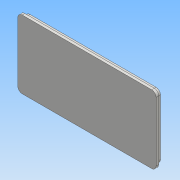
# Autodesk Inventor part: Box2_bottom
Saved by Autodesk Inventor 2016 (Build 200138000, 138)
## iProperties
Created: 2015-09-13
Part Number: Box2_bottom
Material: PPS Plastic
Document SubType Name: Modeling
Designer: Openlab
Density: 1.637 g/cm^3
Appearance: White
Author: Openlab
Autodesk Inventor part; units mm, degrees
ref_plane "YZ Plane" through (0, 0, 0) normal (1, 0, 0) x (0, 1, 0)
ref_plane "XZ Plane" through (0, 0, 0) normal (0, 1, 0) x (-1, 0, 0)
ref_plane "XY Plane" through (0, 0, 0) normal (0, 0, 1) x (1, 0, 0)
sketch "Sketch1" plane through (0, 0, 0) normal (0, 1, 0) x (-1, 0, 0)
  line L0 (-70, 35) -> (70, 35)
  line L1 (75, 30) -> (75, -30)
  line L2 (70, -35) -> (-70, -35)
  line L3 (-75, -30) -> (-75, 30)
  line L4 (-75, 35) -> (75, -35) construction
  line L5 (75, 35) -> (-75, -35) construction
  arc A0 (75, 30) -> (70, 35) centre (70, 30) ccw
  arc A1 (70, -35) -> (75, -30) centre (70, -30) ccw
  arc A2 (-70, 35) -> (-75, 30) centre (-70, 30) ccw
  arc A3 (-75, -30) -> (-70, -35) centre (-70, -30) ccw
  line L6 (-72, 37) -> (72, 37)
  line L7 (77, 32) -> (77, -32)
  line L8 (72, -37) -> (-72, -37)
  line L9 (-77, -32) -> (-77, 32)
  line L10 (-77, 37) -> (77, -37) construction
  line L11 (77, 37) -> (-77, -37) construction
  arc A4 (77, 32) -> (72, 37) centre (72, 32) ccw
  arc A5 (72, -37) -> (77, -32) centre (72, -32) ccw
  arc A6 (-77, -32) -> (-72, -37) centre (-72, -32) ccw
  arc A7 (-72, 37) -> (-77, 32) centre (-72, 32) ccw
  line L12 (74, 39) -> (-74, 39)
  line L13 (-79, 34) -> (-79, -34)
  line L14 (-74, -39) -> (74, -39)
  line L15 (79, -34) -> (79, 34)
  line L16 (79, 39) -> (-79, -39) construction
  line L17 (-79, 39) -> (79, -39) construction
  arc A8 (79, 34) -> (74, 39) centre (74, 34) ccw
  arc A9 (-74, 39) -> (-79, 34) centre (-74, 34) ccw
  arc A10 (-79, -34) -> (-74, -39) centre (-74, -34) ccw
  arc A11 (74, -39) -> (79, -34) centre (74, -34) ccw
  line L18 (-22.75, 23.25) -> (-35.25, 23.25) construction
  line L19 (-35.25, 23.25) -> (-35.25, 19) construction
  line L20 (-35.25, 10.75) -> (-22.75, 10.75) construction
  line L21 (-22.75, 10.75) -> (-22.75, 15) construction
  line L22 (56.9183, 17) -> (21.35, 17) construction
  line L23 (40.8, -24) -> (40.8, -20.1) construction
  line L24 (-55.8, 24) -> (-55.8, 12) construction
  line L25 (-20.25, 15.5) -> (-22.25, 15.5) construction
  line L26 (-22.25, 18.5) -> (-20.25, 18.5) construction
  line L27 (-35.75, 15.5) -> (-37.75, 15.5) construction
  line L28 (-37.75, 18.5) -> (-35.75, 18.5) construction
  line L29 (-40.55, 18.5) -> (-53.5, 18.5) construction
  line L30 (-40.55, 15.5) -> (-53.5, 15.5) construction
  line L31 (-60, 8.5) -> (45, 8.5) construction
  line L32 (38.5, 20.5) -> (37, 20.5) construction
  line L33 (37, 13.5) -> (38.5, 13.5) construction
  line L34 (-60, 5) -> (-60, -25) construction
  line L35 (21.35, -8.5) -> (45, -8.5) construction
  line L36 (-29, 20.0147) -> (-29, -25.5) construction
  line L37 (31.2062, 0) -> (-4.2501, 0) construction
  line L38 (-35.25, 6.25) -> (-35.25, 2) construction
  line L39 (-22.75, 6.25) -> (-35.25, 6.25) construction
  line L40 (-22.75, -6.25) -> (-22.75, -2) construction
  line L41 (-35.25, -6.25) -> (-22.75, -6.25) construction
  line L42 (-22.25, 1.5) -> (-20.25, 1.5) construction
  line L43 (-20.25, -1.5) -> (-22.25, -1.5) construction
  line L44 (38.5, 3.5) -> (37, 3.5) construction
  line L45 (37, -3.5) -> (38.5, -3.5) construction
  line L46 (-22.75, -10.75) -> (-35.25, -10.75) construction
  line L47 (-22.75, -23.25) -> (-22.75, -19) construction
  line L48 (-35.25, -23.25) -> (-22.75, -23.25) construction
  line L49 (56.3008, -17) -> (21.35, -17) construction
  line L50 (38.5, -13.5) -> (37, -13.5) construction
  line L51 (37, -20.5) -> (38.5, -20.5) construction
  line L52 (-20.25, -18.5) -> (-22.25, -18.5) construction
  line L53 (44.5, 5.5) -> (43.5, 5.5) construction
  line L54 (41.3, 11.5) -> (43.5, 11.5) construction
  line L55 (-37.75, -15.5) -> (-35.75, -15.5) construction
  line L56 (-35.75, -18.5) -> (-37.75, -18.5) construction
  line L57 (-40.55, -18.5) -> (-53.5, -18.5) construction
  line L58 (-37.75, 1.5) -> (-35.75, 1.5) construction
  line L59 (-35.75, -1.5) -> (-37.75, -1.5) construction
  line L60 (-40.55, -1.5) -> (-53.5, -1.5) construction
  line L61 (-58.5, 5.5) -> (-59.5, 5.5) construction
  line L62 (-59.5, 11.5) -> (-58.5, 11.5) construction
  line L63 (38.5, 5.5) -> (37, 5.5) construction
  line L64 (37, 5.5) -> (37, 11.5) construction
  line L65 (37, 11.5) -> (38.5, 11.5) construction
  line L66 (-53.5, 5.5) -> (-52.5, 5.5) construction
  line L67 (-52.5, 5.5) -> (-52.5, 11.5) construction
  line L68 (-52.5, 11.5) -> (-53.5, 11.5) construction
  line L69 (-54, 24) -> (-54, 19) construction
  line L70 (-54, 5) -> (-54, 2) construction
  arc A12 (-12.95, 13.5) -> (-12.95, 3.5) centre (-12.95, 8.5) ccw construction
  arc A13 (31, 3.5) -> (31, 13.5) centre (31, 8.5) ccw construction
  arc A14 (-12.95, -3.5) -> (-12.95, -13.5) centre (-12.95, -8.5) ccw construction
  arc A15 (31, -13.5) -> (31, -3.5) centre (31, -8.5) ccw construction
  line L71 (-12.95, 13.5) -> (31, 13.5) construction
  line L72 (-12.95, 3.5) -> (31, 3.5) construction
  line L73 (-12.95, -3.5) -> (31, -3.5) construction
  line L74 (-12.95, -13.5) -> (31, -13.5) construction
  arc A16 (-45.05, -13.5) -> (-45.05, -3.5) centre (-45.05, -8.5) ccw construction
  line L75 (43.5, -24) -> (43.5, -19.6) construction
  line L76 (-58.5, 24) -> (-58.5, 11.5) construction
  arc A17 (-46, -3.5) -> (-46, -13.5) centre (-46, -8.5) ccw construction
  arc A18 (-46, 13.5) -> (-46, 3.5) centre (-46, 8.5) ccw construction
  line L77 (-45.05, -13.5) -> (-46, -13.5) construction
  line L78 (-46, -3.5) -> (-45.05, -3.5) construction
  line L79 (-46, 3.5) -> (-45.05, 3.5) construction
  line L80 (-45.05, 13.5) -> (-46, 13.5) construction
  arc A19 (-45.05, 3.5) -> (-45.05, 13.5) centre (-45.05, 8.5) ccw construction
  line L81 (29.8763, -15.5) -> (-17.45, -15.5) construction
  line L82 (29.8763, -18.5) -> (-17.45, -18.5) construction
  line L83 (29.8763, -1.5) -> (-17.45, -1.5) construction
  line L84 (29.8763, 1.5) -> (-17.45, 1.5) construction
  line L85 (29.8763, 15.5) -> (-17.45, 15.5) construction
  line L86 (29.8763, 18.5) -> (-17.45, 18.5) construction
  arc A20 (32, -14.4) -> (29.8763, -15.5) centre (32, -17) ccw construction
  arc A21 (29.8763, -18.5) -> (32, -19.6) centre (32, -17) ccw construction
  arc A22 (32, 2.6) -> (29.8763, 1.5) centre (32, 0) ccw construction
  arc A23 (29.8763, -1.5) -> (32, -2.6) centre (32, 0) ccw construction
  arc A24 (32, 19.6) -> (29.8763, 18.5) centre (32, 17) ccw construction
  arc A25 (29.8763, 15.5) -> (32, 14.4) centre (32, 17) ccw construction
  arc A26 (34.4725, -25.0625) -> (31, -22) centre (31, -25.5) ccw construction
  arc A27 (-12.95, -22) -> (-16.4225, -25.0625) centre (-12.95, -25.5) ccw construction
  arc A28 (35.7697, -24) -> (31, -20.5) centre (31, -25.5) ccw construction
  line L87 (31, -20.5) -> (-12.95, -20.5) construction
  line L88 (34.9686, -25.5) -> (44.5, -25.5) construction
  line L89 (31, -22) -> (-12.95, -22) construction
  arc A29 (-12.95, -20.5) -> (-17.7197, -24) centre (-12.95, -25.5) ccw construction
  arc A30 (-17.6941, 23.9209) -> (-12.95, 20.5) centre (-12.95, 25.5) ccw construction
  arc A31 (-16.4225, 25.0625) -> (-12.95, 22) centre (-12.95, 25.5) ccw construction
  line L90 (31, 22) -> (-12.95, 22) construction
  line L91 (31, 20.5) -> (-12.95, 20.5) construction
  line L92 (35.7697, 24) -> (40.8, 24) construction
  line L93 (44.5, 25.5) -> (34.9686, 25.5) construction
  arc A32 (31, 22) -> (34.4725, 25.0625) centre (31, 25.5) ccw construction
  arc A33 (31, 20.5) -> (35.7697, 24) centre (31, 25.5) ccw construction
  arc A34 (-41.5775, -25.0625) -> (-45.05, -22) centre (-45.05, -25.5) ccw construction
  arc A35 (-46, -22) -> (-49.4725, -25.0625) centre (-46, -25.5) ccw construction
  line L94 (-45.05, -20.5) -> (-46, -20.5) construction
  line L95 (-45.05, -22) -> (-46, -22) construction
  arc A36 (-46, -20.5) -> (-50.7697, -24) centre (-46, -25.5) ccw construction
  arc A37 (-40.2803, -24) -> (-45.05, -20.5) centre (-45.05, -25.5) ccw construction
  line L96 (-17.7197, -24) -> (-40.2803, -24) construction
  line L97 (-50.7697, -24) -> (-58.5, -24) construction
  line L98 (-59.5, -25.5) -> (-49.9686, -25.5) construction
  line L99 (-17.2197, -25.5) -> (-16.9186, -25.5) construction
  line L100 (-45.05, 20.5) -> (-46, 20.5) construction
  line L101 (-45.05, 22) -> (-46, 22) construction
  arc A38 (-49.4725, 25.0625) -> (-46, 22) centre (-46, 25.5) ccw construction
  arc A39 (-45.05, 22) -> (-41.5775, 25.0625) centre (-45.05, 25.5) ccw construction
  arc A40 (-50.7697, 24) -> (-46, 20.5) centre (-46, 25.5) ccw construction
  arc A41 (-45.05, 20.5) -> (-40.336, 23.8333) centre (-45.05, 25.5) ccw construction
  line L102 (-16.9186, 25.5) -> (-17.2197, 25.5) construction
  line L103 (-49.9686, 25.5) -> (-59.5, 25.5) construction
  line L104 (-58.5, 24) -> (-50.7697, 24) construction
  line L105 (-40.3074, 24) -> (-17.7197, 24) construction
  line L106 (-17.7197, -24) -> (-17.7197, -25) construction
  line L107 (-40.2803, -24) -> (-40.2803, -25) construction
  line L108 (-40.3074, 24) -> (-40.3074, 25) construction
  line L109 (-17.7197, 24.0788) -> (-17.7197, 25) construction
  line L110 (43.5, 11.5) -> (44.5, 11.5) construction
  line L111 (43.5, 5.5) -> (41.3, 5.5) construction
  line L112 (-56.3, 11.5) -> (-58.5, 11.5) construction
  line L113 (-56.3, 5.5) -> (-58.5, 5.5) construction
  line L114 (-17.95, -21) -> (-19.75, -21) construction
  line L115 (-19.75, -13) -> (-17.95, -13) construction
  line L116 (-17.95, -4) -> (-19.75, -4) construction
  line L117 (-19.75, 4) -> (-17.95, 4) construction
  line L118 (-17.95, 13) -> (-19.75, 13) construction
  line L119 (-19.75, 21) -> (-17.95, 21) construction
  line L120 (-38.25, -21) -> (-40.05, -21) construction
  line L121 (-40.05, -13) -> (-38.25, -13) construction
  line L122 (-38.25, -4) -> (-40.05, -4) construction
  line L123 (-40.05, 4) -> (-38.25, 4) construction
  line L124 (-38.25, 13) -> (-40.05, 13) construction
  line L125 (-40.05, 21) -> (-38.25, 21) construction
  line L126 (-17.95, -13) -> (-17.95, -15) construction
  line L127 (-17.95, -19) -> (-17.95, -21) construction
  line L128 (-19.75, -21) -> (-19.75, -19) construction
  line L129 (-17.95, 4) -> (-17.95, 2) construction
  line L130 (-17.95, -2) -> (-17.95, -4) construction
  line L131 (-19.75, -4) -> (-19.75, -2) construction
  line L132 (-19.75, 2) -> (-19.75, 4) construction
  line L133 (-17.95, 21) -> (-17.95, 19) construction
  line L134 (-17.95, 15) -> (-17.95, 13) construction
  line L135 (-19.75, 13) -> (-19.75, 15) construction
  line L136 (-19.75, 19) -> (-19.75, 21) construction
  line L137 (-38.25, -13) -> (-38.25, -15) construction
  line L138 (-38.25, -19) -> (-38.25, -21) construction
  line L139 (-40.05, -21) -> (-40.05, -19) construction
  line L140 (-40.05, -15) -> (-40.05, -13) construction
  line L141 (-38.25, 4) -> (-38.25, 2) construction
  line L142 (-38.25, -2) -> (-38.25, -4) construction
  line L143 (-40.05, -4) -> (-40.05, -2) construction
  line L144 (-40.05, 2) -> (-40.05, 4) construction
  line L145 (-38.25, 21) -> (-38.25, 19) construction
  line L146 (-38.25, 15) -> (-38.25, 13) construction
  line L147 (-40.05, 13) -> (-40.05, 15) construction
  line L148 (-40.05, 19) -> (-40.05, 21) construction
  line L149 (38.5, -11.5) -> (37, -11.5) construction
  line L150 (37, -11.5) -> (37, -5.5) construction
  line L151 (37, -5.5) -> (38.5, -5.5) construction
  line L152 (39, -21) -> (39, -24) construction
  arc A42 (-19.75, -19) -> (-20.25, -18.5) centre (-20.25, -19) ccw construction
  arc A43 (-17.45, -18.5) -> (-17.95, -19) centre (-17.45, -19) ccw construction
  arc A44 (-19.75, -2) -> (-20.25, -1.5) centre (-20.25, -2) ccw construction
  arc A45 (-17.45, -1.5) -> (-17.95, -2) centre (-17.45, -2) ccw construction
  arc A46 (-17.95, 2) -> (-17.45, 1.5) centre (-17.45, 2) ccw construction
  arc A47 (-20.25, 1.5) -> (-19.75, 2) centre (-20.25, 2) ccw construction
  arc A48 (-19.75, 15) -> (-20.25, 15.5) centre (-20.25, 15) ccw construction
  arc A49 (-17.45, 15.5) -> (-17.95, 15) centre (-17.45, 15) ccw construction
  arc A50 (-17.95, 19) -> (-17.45, 18.5) centre (-17.45, 19) ccw construction
  arc A51 (-20.25, 18.5) -> (-19.75, 19) centre (-20.25, 19) ccw construction
  arc A52 (-38.25, 19) -> (-37.75, 18.5) centre (-37.75, 19) ccw construction
  arc A53 (-40.55, 18.5) -> (-40.05, 19) centre (-40.55, 19) ccw construction
  arc A54 (-40.05, 15) -> (-40.55, 15.5) centre (-40.55, 15) ccw construction
  arc A55 (-37.75, 15.5) -> (-38.25, 15) centre (-37.75, 15) ccw construction
  arc A56 (-38.25, 2) -> (-37.75, 1.5) centre (-37.75, 2) ccw construction
  arc A57 (-40.55, 1.5) -> (-40.05, 2) centre (-40.55, 2) ccw construction
  arc A58 (-40.05, -2) -> (-40.55, -1.5) centre (-40.55, -2) ccw construction
  arc A59 (-37.75, -1.5) -> (-38.25, -2) centre (-37.75, -2) ccw construction
  arc A60 (-38.25, -15) -> (-37.75, -15.5) centre (-37.75, -15) ccw construction
  arc A61 (-40.55, -15.5) -> (-40.05, -15) centre (-40.55, -15) ccw construction
  arc A62 (-37.75, -18.5) -> (-38.25, -19) centre (-37.75, -19) ccw construction
  arc A63 (-40.05, -19) -> (-40.55, -18.5) centre (-40.55, -19) ccw construction
  line L153 (36.5, -19.6) -> (32, -19.6) construction
  line L154 (37, -13.5) -> (37, -13.9) construction
  line L155 (32, -14.4) -> (36.5, -14.4) construction
  line L156 (36.5, -2.6) -> (32, -2.6) construction
  line L157 (37, 3.5) -> (37, 3.1) construction
  line L158 (37, -3.1) -> (37, -3.5) construction
  line L159 (32, 2.6) -> (36.5, 2.6) construction
  line L160 (36.5, 14.4) -> (32, 14.4) construction
  line L161 (37, 20.5) -> (37, 20.1) construction
  line L162 (37, 13.9) -> (37, 13.5) construction
  line L163 (32, 19.6) -> (36.5, 19.6) construction
  arc A64 (36.5, -14.4) -> (37, -13.9) centre (36.5, -13.9) ccw construction
  arc A65 (39, -12) -> (38.5, -11.5) centre (38.5, -12) ccw construction
  arc A66 (38.5, -5.5) -> (39, -5) centre (38.5, -5) ccw construction
  arc A67 (39, 5) -> (38.5, 5.5) centre (38.5, 5) ccw construction
  arc A68 (38.5, 11.5) -> (39, 12) centre (38.5, 12) ccw construction
  arc A69 (37, -3.1) -> (36.5, -2.6) centre (36.5, -3.1) ccw construction
  arc A70 (36.5, 2.6) -> (37, 3.1) centre (36.5, 3.1) ccw construction
  arc A71 (37, 13.9) -> (36.5, 14.4) centre (36.5, 13.9) ccw construction
  arc A72 (36.5, 19.6) -> (37, 20.1) centre (36.5, 20.1) ccw construction
  line L164 (43.5, -2.6) -> (43.5, 2.6) construction
  line L165 (43.5, -2.6) -> (41.3, -2.6) construction
  line L166 (37, -20.5) -> (37, -20.1) construction
  arc A73 (37, -20.1) -> (36.5, -19.6) centre (36.5, -20.1) ccw construction
  line L167 (39, -13) -> (39, -12) construction
  line L168 (39, 4) -> (39, 5) construction
  line L169 (39, 21) -> (39, 24) construction
  line L170 (43.5, -19.6) -> (43.5, -14.4) construction
  line L171 (43.5, -19.6) -> (41.3, -19.6) construction
  line L172 (43.5, -24) -> (40.8, -24) construction
  line L173 (40.8, -24) -> (39, -24) construction
  line L174 (39, -24) -> (35.7697, -24) construction
  line L175 (41.3, -14.4) -> (43.5, -14.4) construction
  line L176 (43.5, -14.4) -> (43.5, -2.6) construction
  line L177 (40.8, -13.9) -> (40.8, -3.1) construction
  line L178 (39, -4) -> (39, -5) construction
  line L179 (43.5, 2.6) -> (43.5, 5.5) construction
  line L180 (41.3, 2.6) -> (43.5, 2.6) construction
  line L181 (40.8, 3.1) -> (40.8, 5) construction
  line L182 (43.5, 14.4) -> (43.5, 19.6) construction
  line L183 (43.5, 14.4) -> (41.3, 14.4) construction
  line L184 (45, -25) -> (45, 5) construction
  line L185 (43.5, 19.6) -> (43.5, 24) construction
  line L186 (40.8, 20.1) -> (40.8, 24) construction
  line L187 (41.3, 19.6) -> (43.5, 19.6) construction
  line L188 (43.5, 11.5) -> (43.5, 14.4) construction
  line L189 (40.8, 24) -> (43.5, 24) construction
  line L190 (40.8, 12) -> (40.8, 13.9) construction
  line L191 (39, 13) -> (39, 12) construction
  arc A74 (38.5, -13.5) -> (39, -13) centre (38.5, -13) ccw construction
  arc A75 (39, -4) -> (38.5, -3.5) centre (38.5, -4) ccw construction
  arc A76 (38.5, 3.5) -> (39, 4) centre (38.5, 4) ccw construction
  arc A77 (39, 13) -> (38.5, 13.5) centre (38.5, 13) ccw construction
  arc A78 (38.5, 20.5) -> (39, 21) centre (38.5, 21) ccw construction
  arc A79 (41.3, -19.6) -> (40.8, -20.1) centre (41.3, -20.1) ccw construction
  arc A80 (40.8, -13.9) -> (41.3, -14.4) centre (41.3, -13.9) ccw construction
  arc A81 (41.3, -2.6) -> (40.8, -3.1) centre (41.3, -3.1) ccw construction
  arc A82 (40.8, 3.1) -> (41.3, 2.6) centre (41.3, 3.1) ccw construction
  arc A83 (41.3, 14.4) -> (40.8, 13.9) centre (41.3, 13.9) ccw construction
  arc A84 (40.8, 20.1) -> (41.3, 19.6) centre (41.3, 20.1) ccw construction
  line L192 (40.8, 5.5) -> (40.8, 11.5) construction
  line L193 (-54, 15) -> (-54, 12) construction
  line L194 (-53.5, 1.5) -> (-40.55, 1.5) construction
  line L195 (-54, -2) -> (-54, -15) construction
  line L196 (-54, -19) -> (-54, -24) construction
  line L197 (-53.5, -15.5) -> (-40.55, -15.5) construction
  line L198 (-58.5, 5.5) -> (-58.5, -24) construction
  arc A85 (-54, 19) -> (-53.5, 18.5) centre (-53.5, 19) ccw construction
  arc A86 (-53.5, 15.5) -> (-54, 15) centre (-53.5, 15) ccw construction
  arc A87 (-54, 12) -> (-53.5, 11.5) centre (-53.5, 12) ccw construction
  arc A88 (-53.5, 5.5) -> (-54, 5) centre (-53.5, 5) ccw construction
  arc A89 (-54, 2) -> (-53.5, 1.5) centre (-53.5, 2) ccw construction
  arc A90 (-53.5, -1.5) -> (-54, -2) centre (-53.5, -2) ccw construction
  arc A91 (-54, -15) -> (-53.5, -15.5) centre (-53.5, -15) ccw construction
  arc A92 (-53.5, -18.5) -> (-54, -19) centre (-53.5, -19) ccw construction
  arc A93 (39, -21) -> (38.5, -20.5) centre (38.5, -21) ccw construction
  arc A94 (41.3, 5.5) -> (40.8, 5) centre (41.3, 5) ccw construction
  arc A95 (40.8, 12) -> (41.3, 11.5) centre (41.3, 12) ccw construction
  line L199 (40.8, 5.5) -> (41.3, 5.5) construction
  line L200 (40.8, 11.5) -> (41.3, 11.5) construction
  arc A96 (45, 5) -> (44.5, 5.5) centre (44.5, 5) ccw construction
  line L201 (45, 25) -> (45, 12) construction
  arc A97 (44.5, 11.5) -> (45, 12) centre (44.5, 12) ccw construction
  line L202 (45, 5) -> (45, 12) construction
  arc A98 (-59.5, 5.5) -> (-60, 5) centre (-59.5, 5) ccw construction
  line L203 (-60, 12) -> (-60, 25) construction
  arc A99 (-60, 12) -> (-59.5, 11.5) centre (-59.5, 12) ccw construction
  line L204 (-60, 5) -> (-60, 12) construction
  line L205 (-55.8, -24) -> (-55.8, 5) construction
  arc A100 (-56.3, 11.5) -> (-55.8, 12) centre (-56.3, 12) ccw construction
  arc A101 (-55.8, 5) -> (-56.3, 5.5) centre (-56.3, 5) ccw construction
  line L206 (-55.8, 5.5) -> (-55.8, 11.5) construction
  line L207 (-56.3, 11.5) -> (-55.8, 11.5) construction
  line L208 (-56.3, 5.5) -> (-55.8, 5.5) construction
  arc A102 (44.5, -25.5) -> (45, -25) centre (44.5, -25) ccw construction
  arc A103 (34.4725, -25.0625) -> (34.9686, -25.5) centre (34.9686, -25) ccw construction
  arc A104 (-16.9186, -25.5) -> (-16.4225, -25.0625) centre (-16.9186, -25) ccw construction
  arc A105 (-41.5775, -25.0625) -> (-41.0814, -25.5) centre (-41.0814, -25) ccw construction
  arc A106 (-49.9686, -25.5) -> (-49.4725, -25.0625) centre (-49.9686, -25) ccw construction
  arc A107 (-60, -25) -> (-59.5, -25.5) centre (-59.5, -25) ccw construction
  arc A108 (-59.5, 25.5) -> (-60, 25) centre (-59.5, 25) ccw construction
  arc A109 (-49.4725, 25.0625) -> (-49.9686, 25.5) centre (-49.9686, 25) ccw construction
  arc A110 (-41.0814, 25.5) -> (-41.5775, 25.0625) centre (-41.0814, 25) ccw construction
  arc A111 (-16.4225, 25.0625) -> (-16.9186, 25.5) centre (-16.9186, 25) ccw construction
  arc A112 (34.9686, 25.5) -> (34.4725, 25.0625) centre (34.9686, 25) ccw construction
  arc A113 (45, 25) -> (44.5, 25.5) centre (44.5, 25) ccw construction
  line L209 (-22.75, -19) -> (-22.75, -15) construction
  line L210 (-22.75, -15) -> (-22.75, -10.75) construction
  line L211 (-35.25, -15) -> (-35.25, -19) construction
  line L212 (-35.25, -19) -> (-35.25, -23.25) construction
  arc A114 (-22.25, -18.5) -> (-22.75, -19) centre (-22.25, -19) ccw construction
  arc A115 (-22.75, -15) -> (-22.25, -15.5) centre (-22.25, -15) ccw construction
  arc A116 (-35.25, -19) -> (-35.75, -18.5) centre (-35.75, -19) ccw construction
  arc A117 (-17.95, -15) -> (-17.45, -15.5) centre (-17.45, -15) ccw construction
  line L213 (-19.75, -13) -> (-19.75, -15) construction
  line L214 (-20.25, -15.5) -> (-22.25, -15.5) construction
  arc A118 (-20.25, -15.5) -> (-19.75, -15) centre (-20.25, -15) ccw construction
  line L215 (-35.25, -10.75) -> (-35.25, -15) construction
  arc A119 (-35.75, -15.5) -> (-35.25, -15) centre (-35.75, -15) ccw construction
  line L216 (-22.75, -2) -> (-22.75, 2) construction
  line L217 (-22.75, 2) -> (-22.75, 6.25) construction
  line L218 (-35.25, -2) -> (-35.25, -6.25) construction
  line L219 (-35.25, 2) -> (-35.25, -2) construction
  line L220 (-22.75, 15) -> (-22.75, 19) construction
  line L221 (-22.75, 19) -> (-22.75, 23.25) construction
  line L222 (-35.25, 19) -> (-35.25, 15) construction
  line L223 (-35.25, 15) -> (-35.25, 10.75) construction
  arc A120 (-22.25, -1.5) -> (-22.75, -2) centre (-22.25, -2) ccw construction
  arc A121 (-22.75, 2) -> (-22.25, 1.5) centre (-22.25, 2) ccw construction
  arc A122 (-35.25, -2) -> (-35.75, -1.5) centre (-35.75, -2) ccw construction
  arc A123 (-35.75, 1.5) -> (-35.25, 2) centre (-35.75, 2) ccw construction
  arc A124 (-22.25, 15.5) -> (-22.75, 15) centre (-22.25, 15) ccw construction
  arc A125 (-22.75, 19) -> (-22.25, 18.5) centre (-22.25, 19) ccw construction
  arc A126 (-35.75, 18.5) -> (-35.25, 19) centre (-35.75, 19) ccw construction
  arc A127 (-35.25, 15) -> (-35.75, 15.5) centre (-35.75, 15) ccw construction
  arc A128 (-17.7197, -25) -> (-17.2197, -25.5) centre (-17.2197, -25) ccw construction
  line L224 (-41.0814, -25.5) -> (-40.7803, -25.5) construction
  line L225 (-40.7803, -25.5) -> (-17.2197, -25.5) construction
  arc A129 (-40.7803, -25.5) -> (-40.2803, -25) centre (-40.7803, -25) ccw construction
  arc A130 (-17.2197, 25.5) -> (-17.7197, 25) centre (-17.2197, 25) ccw construction
  line L226 (-41.0814, 25.5) -> (-40.8074, 25.5) construction
  line L227 (-40.8074, 25.5) -> (-17.2197, 25.5) construction
  arc A131 (-40.3074, 25) -> (-40.8074, 25.5) centre (-40.8074, 25) ccw construction
  arc A132 (-17.7197, 24.0788) -> (-17.6941, 23.9209) centre (-17.2197, 24.0788) ccw construction
  arc A133 (-40.336, 23.8333) -> (-40.3074, 24) centre (-40.8074, 24) ccw construction
  line L228 (-23.25, 25.25) -> (-34.75, 25.25)
  line L229 (-37.25, 22.75) -> (-37.25, -22.75)
  line L230 (-34.75, -25.25) -> (-23.25, -25.25)
  line L231 (-20.75, -22.75) -> (-20.75, 22.75)
  line L232 (-20.75, 25.25) -> (-37.25, -25.25) construction
  line L233 (-37.25, 25.25) -> (-20.75, -25.25) construction
  arc A134 (-23.25, -25.25) -> (-20.75, -22.75) centre (-23.25, -22.75) ccw
  arc A135 (-37.25, -22.75) -> (-34.75, -25.25) centre (-34.75, -22.75) ccw
  arc A136 (-20.75, 22.75) -> (-23.25, 25.25) centre (-23.25, 22.75) ccw
  arc A137 (-34.75, 25.25) -> (-37.25, 22.75) centre (-34.75, 22.75) ccw
  line L234 (67, 32) -> (-67, 32)
  line L235 (-72, 27) -> (-72, -27)
  line L236 (-67, -32) -> (67, -32)
  line L237 (72, -27) -> (72, 27)
  line L238 (72, 32) -> (-72, -32) construction
  line L239 (-72, 32) -> (72, -32) construction
  arc A138 (67, -32) -> (72, -27) centre (67, -27) ccw
  arc A139 (-72, -27) -> (-67, -32) centre (-67, -27) ccw
  arc A140 (-67, 32) -> (-72, 27) centre (-67, 27) ccw
  arc A141 (72, 27) -> (67, 32) centre (67, 27) ccw
  line L240 (26.3397, -21.5) -> (-2.6603, -21.5)
  line L241 (-2.6603, -21.5) -> (-2.6603, 21.5)
  line L242 (-2.6603, 21.5) -> (26.3397, 21.5)
  line L243 (26.3397, 21.5) -> (26.3397, -21.5)
  line L244 (26.3397, -21.5) -> (-2.6603, 21.5) construction
  line L245 (-2.6603, -21.5) -> (26.3397, 21.5) construction
  point P0 (0, 0)
  point P1 (0, 0)
  point P2 (0, 0)
  point P3 (-29, -17)
  point P4 (-29, 0)
  point P5 (-29, 17)
  point P6 (43.5, -8.5)
  point P7 (11.8397, 0)
  point P8 (11.8397, 0)
  dimension "d0" = 150
  dimension "d1" = 70
  dimension "d2" = 5
  dimension "d3" = 2
  dimension "d4" = 2
  dimension "d5" = 5
  dimension "d6" = 4
  dimension "d7" = 4
  dimension "d8" = 5
  dimension "d13" = 7
  dimension "d14" = 17
  dimension "d15" = 17
  dimension "d16" = 17
  dimension "d17" = 6
  dimension "d18" = 6
  dimension "d19" = 5
  dimension "d20" = 1.5
  dimension "d21" = 1.5
  dimension "d22" = 1.5
  dimension "d23" = 17
  dimension "d24" = 17
  dimension "d25" = 2.7
  dimension "d26" = 2.7
  dimension "d27" = 6
  dimension "d28" = 25
  dimension "d29" = 5
  dimension "d30" = 1.8
  dimension "d31" = 8
  dimension "d32" = 5
  dimension "d33" = 5
  dimension "d34" = 12.5
  dimension "d35" = 51
  dimension "d36" = 8
  dimension "d37" = 7
  dimension "d38" = 7
  dimension "d39" = 2
  dimension "d40" = 1.8
  dimension "d41" = 8
  dimension "d42" = 1.8
  dimension "d43" = 2.7
  dimension "d44" = 1.5
  dimension "d45" = 3
  dimension "d46" = 3
  dimension "d47" = 3
  dimension "d48" = 0.5
  dimension "d49" = 68
  dimension "d50" = 5.2
  dimension "d51" = 7
  dimension "d52" = 5.2
  dimension "d53" = 5.2
  dimension "d54" = 1.5
  dimension "d55" = 1.5
  dimension "d56" = 0.5
  dimension "d57" = 0.5
  dimension "d58" = 0.5
  dimension "d59" = 6
  dimension "d60" = 0.5
  dimension "d61" = 12.5
  dimension "d62" = 3
  dimension "d63" = 3
  dimension "d64" = 12.5
  dimension "d65" = 12.5
  dimension "d66" = 0.5
  dimension "d67" = 0.5
  constraints: 494 end point, 287 point on circle, 265 tangent, 169 perpendicular, 142 centre point, 124 equal radius, 111 collinear, 81 parallel, 75 point on line, 35 horizontal, 15 midpoint, 14 vertical alignment, 10 coincident, 9 vertical, 7 horizontal alignment, 38 other
  measures "d0" distance of L4.end L5.end
  measures "d1" distance of L5.start L4.end
  measures "d2" radius of A0
  measures "d3" distance between parallel lines of L8 L2
  measures "d4" distance between parallel lines of L7 L1
  measures "d5" radius of A4
  measures "d6" distance between parallel lines of L15 L1
  measures "d7" distance between parallel lines of L14 L2
  measures "d8" radius of A8
  measures "d13" distance of L32.end L33.start
  measures "d14" distance between parallel lines of L37 L22
  measures "d15" distance between parallel lines of L49 L37
  measures "d16" distance between parallel lines of L31 L35
  measures "d17" distance of L63.end L64.end
  measures "d18" distance of L66.end L67.end
  measures "d19" radius of A28
  measures "d20" radial gap between concentric circles of A26 A28
  measures "d21" distance between parallel lines of L93 L92
  measures "d22" distance between parallel lines of L97 L98
  measures "d23" distance between parallel lines of L35 L98
  measures "d24" distance between parallel lines of L103 L31
  measures "d25" distance between parallel lines of L76 L24
  measures "d26" distance between parallel lines of L23 L75
  measures "d27" distance between parallel lines of L111 L54
  measures "d28" distance between parallel lines of L69 L36
  measures "d29" radius of A14
  measures "d30" distance of L114.start L114.end
  measures "d31" distance between parallel lines of L115 L114
  measures "d32" distance from line of A27.centre L127
  measures "d33" distance from line of A37.centre L139
  measures "d34" distance between parallel lines of L18 L20
  measures "d35" distance between parallel lines of L93 L88
  measures "d36" distance from line of A26.centre L152
  measures "d37" distance between parallel lines of L44 L45
  measures "d38" distance between parallel lines of L50 L51
  measures "d39" distance between parallel lines of L64 L168
  measures "d40" distance between parallel lines of L152 L23
  measures "d41" distance from line of L196 A36.centre
  measures "d42" distance between parallel lines of L24 L196
  measures "d43" distance between parallel lines of L198 L24
  measures "d44" distance between parallel lines of L34 L198
  measures "d45" distance between parallel lines of L197 L57
  measures "d46" distance between parallel lines of L60 L194
  measures "d47" distance between parallel lines of L29 L30
  measures "d48" radius of A44
  measures "d49" distance between parallel lines of L169 L36
  measures "d50" distance between parallel lines of L175 L171
  measures "d51" distance from line of A22.centre L178
  measures "d52" distance between parallel lines of L180 L165
  measures "d53" distance between parallel lines of L187 L183
  measures "d54" distance between parallel lines of L70 L67
  measures "d55" distance between parallel lines of L75 L184
  measures "d56" radius of A94
  measures "d57" radius of A96
  measures "d58" radius of A97
  measures "d59" distance between parallel lines of L62 L61
  measures "d60" radius of A102
  measures "d61" distance between parallel lines of L46 L48
  measures "d62" distance between parallel lines of L47 L128
  measures "d63" distance between parallel lines of L138 L212
  measures "d64" distance between parallel lines of L39 L41
  measures "d65" distance between parallel lines of L223 L21
  measures "d66" radius of A128
  measures "d67" radius of A129
extrude "Extrusion1" add sketch "Sketch1" along normal blind 7 contours L0 A0 L1 A1 L2 A3 L3 A2 | L6 A4 L7 A5 L8 A6 L9 A7
extrude "Extrusion2" add sketch "Sketch1" along normal blind 3 contours A8 L15 A11 L14 A10 L13 A9 L12
extrude "Extrusion3" add sketch "Sketch1" along normal blind 2.5 contours A136 L231 A134 L230 A135 L229 A137 L228 | A141 L237 A138 L236 A139 L235 A140 L234 | L240 L241 L242 L243
body "Solid1"
